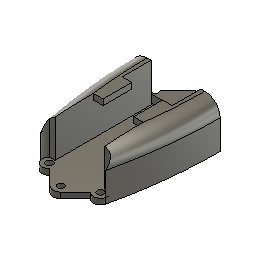
Tail (9V holder) (Autodesk Fusion 360 design; units mm, degrees)
Autodesk Fusion 360 part; units mm, degrees
sketch "9V Holder Sketch" plane through (0, 0, 0) normal (0, 1, 0) x (1, 0, 0)
  line L0 (16, -25) -> (-16, -25)
  line L1 (-16, -25) -> (-16, 25)
  line L2 (-16, 25) -> (16, 25)
  line L3 (16, 25) -> (16, -25)
  line L4 (16, -25) -> (-16, 25) construction
  line L5 (-16, -25) -> (16, 25) construction
  circle A0 centre (0, 35) radius 1.7
  circle A1 centre (0, 35) radius 4
  line L6 (16, 25) -> (2.7909, 37.8655)
  line L7 (-16, 25) -> (-2.7909, 37.8655)
  line L8 (13, 25) -> (13, -25)
  line L9 (-13, 25) -> (-13, -25)
  line L10 (13, 10) -> (8, 10)
  line L11 (8, 10) -> (8, -5)
  line L12 (8, -5) -> (13, -5)
  line L13 (-13, 10) -> (-8, 10)
  line L14 (-8, 10) -> (-8, -5)
  line L15 (-8, -5) -> (-13, -5)
  line L16 (-10.3531, 30.5) -> (10.3531, 30.5)
  circle A2 centre (0, -35) radius 4
  circle A3 centre (0, -35) radius 1.7
  line L17 (2.7909, -37.8655) -> (16, -25)
  line L18 (-2.7909, -37.8655) -> (-16, -25)
  arc A4 (4.2677, -36.4271) -> (-4.2677, -36.4271) centre (0, -35) ccw
  line L19 (10.3531, -30.5) -> (-10.3531, -30.5)
  arc A5 (-4.2677, 36.4271) -> (4.2677, 36.4271) centre (0, 35) ccw
  arc A6 (16, 25) -> (10.6273, 30.233) centre (13.3136, 27.6165) ccw
  circle A7 centre (13.3136, 27.6165) radius 1.75
  arc A8 (-10.6273, 30.233) -> (-16, 25) centre (-13.3136, 27.6165) ccw
  arc A9 (-16, -25) -> (-10.6273, -30.233) centre (-13.3136, -27.6165) ccw
  arc A10 (10.6273, -30.233) -> (16, -25) centre (13.3136, -27.6165) ccw
  circle A11 centre (-13.3136, -27.6165) radius 1.75
  circle A12 centre (13.3136, -27.6165) radius 1.75
  circle A13 centre (-13.3136, 27.6165) radius 1.75
  line L20 (-16, 25) -> (-23, 25)
  arc A14 (-23, 25) -> (-16.9694, -28.452) centre (216.8991, 25) ccw
  line L21 (-23, 25) -> (-23, 27) construction
  line L22 (16, 25) -> (23, 25)
  line L23 (23, 25) -> (23, 31.9603) construction
  arc A15 (16.9694, -28.452) -> (23, 25) centre (-216.8991, 25) ccw
  line L24 (13.3136, 25.8665) -> (16.6303, 25.8665)
  line L25 (13.3136, 25.8665) -> (13.3136, 25)
  line L26 (-13.3136, 25.8665) -> (-13.3136, 25)
  line L27 (-13.3136, 25.8665) -> (-16.6303, 25.8665)
  arc A16 (-11.2918, 30.7747) -> (-10.3531, 30.5) centre (-10.3531, 32.241) ccw
  arc A17 (10.3531, 30.5) -> (11.2918, 30.7747) centre (10.3531, 32.241) ccw
  dimension "d94" = 32
  dimension "d95" = 50
  dimension "d96" = 3.4
  dimension "d97" = 8
  dimension "d98" = 10
  dimension "d99" = 3
  dimension "d100" = 3
  dimension "d111" = 15
  dimension "d112" = 5
  dimension "d113" = 5
  dimension "d116" = 0.5
  dimension "d232" = 8
  dimension "d233" = 3.4
  dimension "d234" = 10
  dimension "d236" = 0.5
  dimension "d237" = 3.5
  dimension "d238" = 2
  dimension "d239" = 3.5
  dimension "d240" = 3.5
  dimension "d241" = 3.5
  dimension "d243" = 2
  dimension "d244" = 2
  dimension "d245" = 2
  dimension "d465" = 7
  dimension "d477" = 7
  dimension "d583" = 15
  constraint horizontal L0
  constraint perpendicular L0 L1
  constraint parallel L0 L2
  constraint parallel L1 L3
  constraint coincident L4 origin
  constraint coincident L5 origin
  constraint concentric A0 A1
  constraint coincident A1 L6.end
  constraint coincident A1 L7.end
  constraint tangent A1 L7
  constraint tangent A1 L6
  constraint vertical origin A0.centre
  constraint coincident L2 L8.start
  constraint coincident L0 L8.end
  constraint perpendicular L0 L8
  constraint coincident L2 L9.start
  constraint coincident L0 L9.end
  constraint perpendicular L0 L9
  constraint coincident L8 L10.start
  constraint perpendicular L8 L10
  constraint perpendicular L10 L11
  constraint coincident L8 L12.end
  constraint perpendicular L8 L12
  constraint coincident L9 L13.start
  constraint perpendicular L9 L13
  constraint perpendicular L13 L14
  constraint coincident L9 L15.end
  constraint perpendicular L9 L15
  constraint collinear L10 L13
  constraint collinear L12 L15
  constraint concentric A0 A5
  constraint horizontal L16
  constraint coincident L7 L16.start
  constraint coincident L6 L16.end
  constraint tangent L16 A5
  constraint concentric A2 A3
  constraint coincident A2 L17.start
  constraint coincident A2 L18.start
  constraint vertical origin A2.centre
  constraint tangent A2 L17
  constraint tangent A2 L18
  constraint concentric A2 A4
  constraint coincident L18 A4.end
  constraint coincident L17 A4.start
  constraint coincident L17 L19.start
  constraint coincident L18 L19.end
  constraint horizontal L19
  constraint tangent A4 L19
  constraint coincident L6 A5.end
  constraint coincident L7 A5.start
  constraint coincident L6 A6.centre
  constraint concentric A6 A7
  constraint coincident L6 A6.end
  constraint coincident L7 A8.centre
  constraint coincident L18 A9.centre
  constraint coincident L17 A10.centre
  constraint concentric A9 A11
  constraint concentric A10 A12
  constraint concentric A8 A13
  constraint coincident L7 A8.start
  constraint coincident L18 A9.end
  constraint coincident L17 A10.start
  constraint coincident L1 L2.start
  constraint perpendicular L1 L20
  constraint tangent A9 A14
  constraint coincident A9 A14.end
  constraint perpendicular L20 L21
  constraint tangent A14 L21
  constraint coincident L1.end L2.start
  constraint perpendicular L3 L22
  constraint perpendicular L22 L23
  constraint coincident A10 A15.start
  constraint tangent A10 A15
  constraint tangent L23 A15
  constraint coincident A7 L24.start
  constraint horizontal L24
  constraint coincident L2 L25.end
  constraint perpendicular L2 L25
  constraint tangent A7 L24
  constraint coincident A6 L24.end
  constraint coincident A13 L26.start
  constraint coincident L2 L26.end
  constraint perpendicular L2 L26
  constraint perpendicular L26 L27
  constraint coincident A8 L27.end
  constraint tangent A13 L27
  constraint coincident A8 A16.start
  constraint tangent L16 A16
  constraint tangent A8 A16
  constraint coincident A6 A17.end
  constraint tangent A6 A17
  constraint tangent L16 A17
  measures "d94" distance of L1.end L2.end
  measures "d95" distance of L0.end L1.end
  measures "d96" diameter of A0
  measures "d97" diameter of A1
  measures "d98" distance of L2 A0.centre
  measures "d99" distance of L1 L9
  measures "d100" distance of L3 L8
  measures "d111" distance of L10 L12
  measures "d112" distance of L8 L11
  measures "d113" distance of L9 L14
  measures "d116" distance of A1 A5
  measures "d232" diameter of A2
  measures "d233" diameter of A3
  measures "d234" distance of L0 A2.centre
  measures "d236" distance of A2 A4
  measures "d237" diameter of A7
  measures "d238" distance of A6 A7
  measures "d239" diameter of A11
  measures "d240" diameter of A12
  measures "d241" diameter of A13
  measures "d243" distance of A8 A13
  measures "d244" distance of A9 A11
  measures "d245" distance of A10 A12
  measures "d465" distance of L1.end L20.end
  measures "d477" distance of L2.end L22.end
  measures "d583" distance of L2 L10
extrude "Extrude1" add sketch "9V Holder Sketch" against normal blind 4 contours L0 L17 L18 L19 A11 A12 | L0 L2 L3 L8 | L17 A10 A12 | L3 A10 L22 A15 | L0 L2 L8 L9 L10 L11 L12 L13 L14 L15 | L0 L1 L2 L9 | L8 L10 L11 L12 | L2 L6 L7 L16 A7 A13 L25 L26 | L6 A6 A7 L24 | L1 A9 L20 A14 | L18 A9 A11 | L9 L13 L14 L15 | L6 A6 A17 | L17 A4 L19 | A2 L17 L18 A4 | L18 A4 L19 | L7 A8 A13 L27 | A2 | L7 A8 A16
extrude "Extrude5" cut 1 faces at (4.4379, 0, -13.0324) along direction (0, -1, 0) blind 1
extrude "Extrude2" add sketch "9V Holder Sketch" along normal blind 20.2 from surface at -1 contours L0 L2 L3 L8 | L3 A10 L22 A15 | L0 L1 L2 L9 | L1 A9 L20 A14
extrude "Extrude4" add sketch "9V Holder Sketch" against normal blind 3 from surface at 19.2 contours L8 L10 L11 L12 | L9 L13 L14 L15
extrude "Extrude3" add sketch "9V Holder Sketch" along normal blind 4 contours L2 L6 L7 L16 A7 A13 L25 L26 | L6 L16 A5 | A1 L6 L7 A5 | L7 L16 A5 | A1
fillet "Fillet3" radius 8 2 edges at (-21.4876, 19.2, 1.8956) (21.4876, 19.2, 1.8956)
equation "d96 = hingeBoltDia + 0.4 mm"
equation "d97 = strutsWidth"
equation "d107 = -frameThickness"
equation "d109 = 17.2 mm + 3 mm"
equation "d118 = frameThickness"
equation "d232 = strutsWidth"
equation "d233 = hingeBoltDia + 0.4 mm"
equation "d237 = rubberbandHole"
equation "d239 = rubberbandHole"
equation "d240 = rubberbandHole"
equation "d241 = rubberbandHole"
equation "hingeBoltDia = 3 mm"
equation "strutsWidth = 8 mm"
equation "frameThickness = 4 mm"
equation "rubberbandHole = 3.5 mm"
named bodies: "9V Holder"
